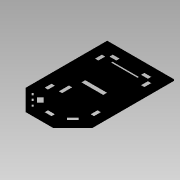
# Autodesk Inventor part: Base Kepala
Saved by Autodesk Inventor 2015 SP1 (Build 190203100, 203)
## iProperties
Created: 2015-02-13
Part Number: Base Kepala
Material: Generic
Document SubType Name: Modeling
Designer: Rafi Kurnia Putra
Density: 1 g/cm^3
Appearance: Default(1)
Author: Rafi Kurnia Putra
Autodesk Inventor part; units mm, degrees
ref_plane "YZ Plane" through (0, 0, 0) normal (1, 0, 0) x (0, 1, 0)
ref_plane "XZ Plane" through (0, 0, 0) normal (0, 1, 0) x (-1, 0, 0)
ref_plane "XY Plane" through (0, 0, 0) normal (0, 0, 1) x (1, 0, 0)
sketch "Sketch1" plane through (0, 0, 0) normal (0, 1, 0) x (-1, 0, 0)
  line L0 (31.6823, -78.8894) -> (44.0567, -66.5151)
  line L1 (24.6113, -71.8184) -> (31.6823, -78.8894)
  line L2 (36.9856, -59.444) -> (24.6113, -71.8184)
  line L3 (44.0567, -66.5151) -> (36.9856, -59.444)
  line L4 (8.75, -88.3884) -> (8.75, -78.3884)
  line L5 (-8.75, -88.3884) -> (8.75, -88.3884)
  line L6 (8.75, -78.3884) -> (-8.75, -78.3884)
  line L7 (-8.75, -78.3884) -> (-8.75, -88.3884)
  line L8 (-31.6827, -78.8894) -> (-24.6116, -71.8184)
  line L9 (-24.6116, -71.8184) -> (-36.986, -59.444)
  line L10 (-44.057, -66.5151) -> (-31.6827, -78.8894)
  line L11 (-36.986, -59.444) -> (-44.057, -66.5151)
  line L12 (-53.5557, -43.5826) -> (-43.5557, -43.5826)
  line L13 (-43.5557, -43.5826) -> (-43.5557, -26.0826)
  line L14 (-43.5557, -26.0826) -> (-53.5557, -26.0826)
  line L15 (-53.5557, -26.0826) -> (-53.5557, -43.5826)
  line L16 (-53.556, 80.1674) -> (-53.556, 62.6674)
  line L17 (-43.556, 80.1674) -> (-53.556, 80.1674)
  line L18 (-43.556, 62.6674) -> (-43.556, 80.1674)
  line L19 (-53.556, 62.6674) -> (-43.556, 62.6674)
  line L20 (-42.0848, 91.6386) -> (-42.0848, 81.6386)
  line L21 (-42.0848, 81.6386) -> (-24.5848, 81.6386)
  line L22 (-24.5848, 81.6386) -> (-24.5848, 91.6386)
  line L23 (-24.5848, 91.6386) -> (-42.0848, 91.6386)
  line L24 (42.0848, 91.6386) -> (24.5848, 91.6386)
  line L25 (42.0848, 81.6386) -> (42.0848, 91.6386)
  line L26 (24.5848, 81.6386) -> (42.0848, 81.6386)
  line L27 (24.5848, 91.6386) -> (24.5848, 81.6386)
  line L28 (43.556, 80.1674) -> (43.556, 62.6674)
  line L29 (53.556, 80.1674) -> (43.556, 80.1674)
  line L30 (53.556, 62.6674) -> (53.556, 80.1674)
  line L31 (43.556, 62.6674) -> (53.556, 62.6674)
  circle A0 centre (37.593, 75.6756) radius 1.75
  circle A1 centre (32.8575, 75.4371) radius 1.75
  circle A2 centre (50.5965, 88.6786) radius 1.75
  line L32 (29.3575, 78.4256) -> (-29.3575, 78.4256)
  line L33 (29.3575, 72.4486) -> (29.3575, 78.4256)
  line L34 (-29.3575, 72.4486) -> (29.3575, 72.4486)
  line L35 (-29.3575, 78.4256) -> (-29.3575, 72.4486)
  circle A3 centre (-32.8575, 75.4371) radius 1.75
  circle A4 centre (-37.593, 75.6756) radius 1.75
  circle A5 centre (-50.5965, 88.6786) radius 1.75
  line L36 (-24.5, 4.9331) -> (24.5, 4.9331)
  circle A6 centre (28, 4.9331) radius 1.75
  circle A7 centre (32.442, 26.7171) radius 1.5
  circle A8 centre (38, 31.4596) radius 1.75
  circle A9 centre (50.5965, 18.9376) radius 1.75
  circle A10 centre (32.4485, 53.6756) radius 1.75
  circle A11 centre (-32.4355, 53.6756) radius 1.75
  circle A12 centre (-50.5965, 18.9376) radius 1.75
  circle A13 centre (-32.442, 26.7171) radius 1.5
  circle A14 centre (-28, 4.9331) radius 1.75
  line L37 (-22.2, -10.9442) -> (-32, -10.9442)
  line L38 (-22.2, -35.1896) -> (-22.2, -10.9442)
  line L39 (-32, -35.1896) -> (-22.2, -35.1896)
  line L40 (-32, -10.9442) -> (-32, -35.1896)
  circle A15 centre (-49.906, -55.5042) radius 1.75
  circle A16 centre (-37.593, -48.9392) radius 1.75
  circle A17 centre (-20, -65.0669) radius 1.75
  circle A18 centre (13.2193, -19.3896) radius 1.75
  circle A19 centre (13.2193, -43.7996) radius 1.75
  circle A20 centre (20, -65.0669) radius 1.75
  circle A21 centre (37.593, -48.9392) radius 1.75
  circle A22 centre (39.7053, -43.7996) radius 1.75
  circle A23 centre (39.7053, -19.3896) radius 1.75
  circle A24 centre (49.9057, -55.5042) radius 1.75
  line L41 (43.5557, -43.5826) -> (53.5557, -43.5826)
  line L42 (43.5557, -26.0826) -> (43.5557, -43.5826)
  line L43 (53.5557, -26.0826) -> (43.5557, -26.0826)
  line L44 (53.5557, -43.5826) -> (53.5557, -26.0826)
  line L45 (24.5, 4.9331) -> (24.5, 15.9376)
  line L46 (24.5, 15.9376) -> (-24.5, 15.9376)
  line L47 (-24.5, 15.9376) -> (-24.5, 4.9331)
  circle A25 centre (14, 31.4596) radius 1.75
  circle A26 centre (-27.94, -53.8096) radius 1.75
  circle A27 centre (20.32, -47.4596) radius 1.75
  line L48 (70.4053, -63.9933) -> (29.1627, -105.2363)
  line L49 (29.1627, -105.2363) -> (-29.1634, -105.2362)
  line L50 (-29.1634, -105.2362) -> (-70.4063, -63.9936)
  line L51 (-70.4063, -63.9936) -> (-70.4063, 108.2408)
  line L52 (-70.4063, 108.2408) -> (70.4053, 108.2411)
  line L53 (70.4053, 108.2411) -> (70.4053, -63.9933)
  line L54 (37.7622, -79.6663) -> (44.8333, -72.5952)
  line L55 (44.8333, -72.5952) -> (46.9546, -74.7165)
  line L56 (46.9546, -74.7165) -> (39.8835, -81.7876)
  line L57 (39.8835, -81.7876) -> (37.7622, -79.6663)
  line L58 (37.7622, -79.6663) -> (46.9546, -74.7165) construction
  line L59 (44.8333, -72.5952) -> (39.8835, -81.7876) construction
  line L60 (34.2266, -83.2018) -> (27.1556, -90.2729)
  line L61 (27.1556, -90.2729) -> (29.2769, -92.3942)
  line L62 (29.2769, -92.3942) -> (36.348, -85.3231)
  line L63 (36.348, -85.3231) -> (34.2266, -83.2018)
  line L64 (34.2266, -83.2018) -> (29.2769, -92.3942) construction
  line L65 (27.1556, -90.2729) -> (36.348, -85.3231) construction
  line L66 (55.4401, -61.9888) -> (48.369, -69.0599)
  line L67 (48.369, -69.0599) -> (50.4903, -71.1812)
  line L68 (50.4903, -71.1812) -> (57.5614, -64.1101)
  line L69 (57.5614, -64.1101) -> (55.4401, -61.9888)
  line L70 (55.4401, -61.9888) -> (50.4903, -71.1812) construction
  line L71 (48.369, -69.0599) -> (57.5614, -64.1101) construction
  line L72 (5, -93.2363) -> (15, -93.2363) construction
  line L73 (-10, -93.2363) -> (-20, -93.2363)
  line L74 (-20, -93.2363) -> (-20, -96.2363)
  line L75 (-20, -96.2363) -> (-10, -96.2363)
  line L76 (-10, -96.2363) -> (-10, -93.2363)
  line L77 (-10, -93.2363) -> (-20, -96.2363) construction
  line L78 (-20, -93.2363) -> (-10, -96.2363) construction
  line L79 (-10, -93.2363) -> (0, -93.2363) construction
  line L80 (20, -96.237) -> (10, -96.237)
  line L81 (10, -96.237) -> (10, -93.237)
  line L82 (10, -93.237) -> (20, -93.237)
  line L83 (20, -93.237) -> (20, -96.237)
  line L84 (20, -96.237) -> (10, -93.237) construction
  line L85 (10, -96.237) -> (20, -93.237) construction
  line L86 (61.4053, 25.443) -> (61.4053, 10.443)
  line L87 (61.4053, 10.443) -> (58.4053, 10.443)
  line L88 (58.4053, 10.443) -> (58.4053, 25.443)
  line L89 (58.4053, 25.443) -> (61.4053, 25.443)
  line L90 (61.4053, 25.443) -> (58.4053, 10.443) construction
  line L91 (61.4053, 10.443) -> (58.4053, 25.443) construction
  line L92 (-37.8487, -79.5805) -> (-44.9198, -72.5095)
  line L93 (-44.9198, -72.5095) -> (-47.0411, -74.6308)
  line L94 (-47.0411, -74.6308) -> (-39.97, -81.7018)
  line L95 (-39.97, -81.7018) -> (-37.8487, -79.5805)
  line L96 (-37.8487, -79.5805) -> (-47.0411, -74.6308) construction
  line L97 (-34.3131, -83.116) -> (-27.242, -90.1871)
  line L98 (-27.242, -90.1871) -> (-29.3633, -92.3084)
  line L99 (-29.3633, -92.3084) -> (-36.4344, -85.2374)
  line L100 (-36.4344, -85.2374) -> (-34.3131, -83.116)
  line L101 (-34.3131, -83.116) -> (-29.3633, -92.3084) construction
  line L102 (-27.242, -90.1871) -> (-36.4344, -85.2374) construction
  line L103 (-55.5071, -61.8836) -> (-48.4359, -68.9546)
  line L104 (-48.4359, -68.9546) -> (-50.5766, -71.0953)
  line L105 (-50.5766, -71.0953) -> (-57.6477, -64.0243)
  line L106 (-57.6477, -64.0243) -> (-55.5071, -61.8836)
  line L107 (-55.5071, -61.8836) -> (-50.5766, -71.0953) construction
  line L108 (-48.4359, -68.9546) -> (-57.6477, -64.0243) construction
  line L109 (61.4053, -7.057) -> (61.4053, -22.057)
  line L110 (61.4053, -22.057) -> (58.4053, -22.057)
  line L111 (58.4053, -22.057) -> (58.4053, -7.057)
  line L112 (58.4053, -7.057) -> (61.4053, -7.057)
  line L113 (61.4053, -7.057) -> (58.4053, -22.057) construction
  line L114 (61.4053, -22.057) -> (58.4053, -7.057) construction
  line L115 (61.4053, -39.557) -> (61.4053, -54.557)
  line L116 (61.4053, -54.557) -> (58.4053, -54.557)
  line L117 (58.4053, -54.557) -> (58.4053, -39.557)
  line L118 (58.4053, -39.557) -> (61.4053, -39.557)
  line L119 (61.4053, -39.557) -> (58.4053, -54.557) construction
  line L120 (61.4053, -54.557) -> (58.4053, -39.557) construction
  line L121 (61.4053, 57.943) -> (61.4053, 42.943)
  line L122 (61.4053, 42.943) -> (58.4053, 42.943)
  line L123 (58.4053, 42.943) -> (58.4053, 57.943)
  line L124 (58.4053, 57.943) -> (61.4053, 57.943)
  line L125 (61.4053, 57.943) -> (58.4053, 42.943) construction
  line L126 (61.4053, 42.943) -> (58.4053, 57.943) construction
  line L127 (61.4053, 25.443) -> (61.4053, 10.443)
  line L128 (61.4053, 10.443) -> (58.4053, 10.443)
  line L129 (58.4053, 10.443) -> (58.4053, 25.443)
  line L130 (58.4053, 25.443) -> (61.4053, 25.443)
  line L131 (61.4053, 25.443) -> (58.4053, 10.443) construction
  line L132 (61.4053, 10.443) -> (58.4053, 25.443) construction
  line L133 (61.4053, -7.057) -> (61.4053, -22.057)
  line L134 (61.4053, -22.057) -> (58.4053, -22.057)
  line L135 (58.4053, -22.057) -> (58.4053, -7.057)
  line L136 (58.4053, -7.057) -> (61.4053, -7.057)
  line L137 (61.4053, -7.057) -> (58.4053, -22.057) construction
  line L138 (61.4053, -22.057) -> (58.4053, -7.057) construction
  line L139 (61.4053, 90.443) -> (61.4053, 75.443)
  line L140 (61.4053, 75.443) -> (58.4053, 75.443)
  line L141 (58.4053, 75.443) -> (58.4053, 90.443)
  line L142 (58.4053, 90.443) -> (61.4053, 90.443)
  line L143 (61.4053, 90.443) -> (58.4053, 75.443) construction
  line L144 (61.4053, 75.443) -> (58.4053, 90.443) construction
  line L145 (61.4053, 57.943) -> (61.4053, 42.943)
  line L146 (61.4053, 42.943) -> (58.4053, 42.943)
  line L147 (58.4053, 42.943) -> (58.4053, 57.943)
  line L148 (58.4053, 57.943) -> (61.4053, 57.943)
  line L149 (61.4053, 57.943) -> (58.4053, 42.943) construction
  line L150 (61.4053, 42.943) -> (58.4053, 57.943) construction
  line L151 (61.4053, 25.443) -> (61.4053, 10.443)
  line L152 (61.4053, 10.443) -> (58.4053, 10.443)
  line L153 (58.4053, 10.443) -> (58.4053, 25.443)
  line L154 (58.4053, 25.443) -> (61.4053, 25.443)
  line L155 (61.4053, 25.443) -> (58.4053, 10.443) construction
  line L156 (61.4053, 10.443) -> (58.4053, 25.443) construction
  line L157 (0, 0) -> (0, -22.057) construction
  line L158 (-61.4053, 25.443) -> (-61.4053, 10.443)
  line L159 (-61.4053, 10.443) -> (-58.4053, 10.443)
  line L160 (-58.4053, 10.443) -> (-58.4053, 25.443)
  line L161 (-58.4053, 25.443) -> (-61.4053, 25.443)
  line L162 (-61.4053, 25.443) -> (-58.4053, 10.443) construction
  line L163 (-61.4053, 10.443) -> (-58.4053, 25.443) construction
  line L164 (-58.4053, -7.057) -> (-61.4053, -7.057)
  line L165 (-58.4053, -22.057) -> (-58.4053, -7.057)
  line L166 (-61.4053, -22.057) -> (-58.4053, -22.057)
  line L167 (-61.4053, -7.057) -> (-61.4053, -22.057)
  line L168 (-61.4053, -7.057) -> (-58.4053, -22.057) construction
  line L169 (-61.4053, -22.057) -> (-58.4053, -7.057) construction
  line L170 (-58.4053, -39.557) -> (-61.4053, -39.557)
  line L171 (-58.4053, -54.557) -> (-58.4053, -39.557)
  line L172 (-61.4053, -54.557) -> (-58.4053, -54.557)
  line L173 (-61.4053, -39.557) -> (-61.4053, -54.557)
  line L174 (-61.4053, -39.557) -> (-58.4053, -54.557) construction
  line L175 (-61.4053, -54.557) -> (-58.4053, -39.557) construction
  line L176 (-58.4053, 57.943) -> (-61.4053, 57.943)
  line L177 (-58.4053, 42.943) -> (-58.4053, 57.943)
  line L178 (-61.4053, 42.943) -> (-58.4053, 42.943)
  line L179 (-61.4053, 57.943) -> (-61.4053, 42.943)
  line L180 (-61.4053, 57.943) -> (-58.4053, 42.943) construction
  line L181 (-61.4053, 42.943) -> (-58.4053, 57.943) construction
  line L182 (-58.4053, 25.443) -> (-61.4053, 25.443)
  line L183 (-58.4053, 10.443) -> (-58.4053, 25.443)
  line L184 (-61.4053, 10.443) -> (-58.4053, 10.443)
  line L185 (-61.4053, 25.443) -> (-61.4053, 10.443)
  line L186 (-61.4053, 25.443) -> (-58.4053, 10.443) construction
  line L187 (-61.4053, 10.443) -> (-58.4053, 25.443) construction
  line L188 (-58.4053, -7.057) -> (-61.4053, -7.057)
  line L189 (-58.4053, -22.057) -> (-58.4053, -7.057)
  line L190 (-61.4053, -22.057) -> (-58.4053, -22.057)
  line L191 (-61.4053, -7.057) -> (-61.4053, -22.057)
  line L192 (-61.4053, -7.057) -> (-58.4053, -22.057) construction
  line L193 (-61.4053, -22.057) -> (-58.4053, -7.057) construction
  line L194 (-58.4053, 90.443) -> (-61.4053, 90.443)
  line L195 (-58.4053, 75.443) -> (-58.4053, 90.443)
  line L196 (-61.4053, 75.443) -> (-58.4053, 75.443)
  line L197 (-61.4053, 90.443) -> (-61.4053, 75.443)
  line L198 (-61.4053, 90.443) -> (-58.4053, 75.443) construction
  line L199 (-61.4053, 75.443) -> (-58.4053, 90.443) construction
  line L200 (-58.4053, 57.943) -> (-61.4053, 57.943)
  line L201 (-58.4053, 42.943) -> (-58.4053, 57.943)
  line L202 (-61.4053, 42.943) -> (-58.4053, 42.943)
  line L203 (-61.4053, 57.943) -> (-61.4053, 42.943)
  line L204 (-61.4053, 57.943) -> (-58.4053, 42.943) construction
  line L205 (-61.4053, 42.943) -> (-58.4053, 57.943) construction
  line L206 (-58.4053, 25.443) -> (-61.4053, 25.443)
  line L207 (-58.4053, 10.443) -> (-58.4053, 25.443)
  line L208 (-61.4053, 10.443) -> (-58.4053, 10.443)
  line L209 (-61.4053, 25.443) -> (-61.4053, 10.443)
  line L210 (-61.4053, 25.443) -> (-58.4053, 10.443) construction
  line L211 (-61.4053, 10.443) -> (-58.4053, 25.443) construction
  line L212 (-7.5214, 96.2408) -> (7.4786, 96.2408)
  line L213 (7.4786, 96.2408) -> (7.4786, 99.2408)
  line L214 (7.4786, 99.2408) -> (-7.5214, 99.2408)
  line L215 (-7.5214, 99.2408) -> (-7.5214, 96.2408)
  line L216 (-7.5214, 96.2408) -> (7.4786, 99.2408) construction
  line L217 (7.4786, 96.2408) -> (-7.5214, 99.2408) construction
  line L218 (-30.5214, 96.2408) -> (-15.5214, 96.2408)
  line L219 (-15.5214, 96.2408) -> (-15.5214, 99.2408)
  line L220 (-15.5214, 99.2408) -> (-30.5214, 99.2408)
  line L221 (-30.5214, 99.2408) -> (-30.5214, 96.2408)
  line L222 (-30.5214, 96.2408) -> (-15.5214, 99.2408) construction
  line L223 (-15.5214, 96.2408) -> (-30.5214, 99.2408) construction
  line L224 (-53.5214, 96.2407) -> (-38.5214, 96.2407)
  line L225 (-38.5214, 96.2407) -> (-38.5214, 99.2407)
  line L226 (-38.5214, 99.2407) -> (-53.5214, 99.2407)
  line L227 (-53.5214, 99.2407) -> (-53.5214, 96.2407)
  line L228 (-53.5214, 96.2407) -> (-38.5214, 99.2407) construction
  line L229 (-38.5214, 96.2407) -> (-53.5214, 99.2407) construction
  line L230 (15.4786, 96.2409) -> (30.4786, 96.2409)
  line L231 (30.4786, 96.2409) -> (30.4786, 99.2409)
  line L232 (30.4786, 99.2409) -> (15.4786, 99.2409)
  line L233 (15.4786, 99.2409) -> (15.4786, 96.2409)
  line L234 (15.4786, 96.2409) -> (30.4786, 99.2409) construction
  line L235 (30.4786, 96.2409) -> (15.4786, 99.2409) construction
  line L236 (-7.5214, 96.2408) -> (7.4786, 96.2408)
  line L237 (7.4786, 96.2408) -> (7.4786, 99.2408)
  line L238 (7.4786, 99.2408) -> (-7.5214, 99.2408)
  line L239 (-7.5214, 99.2408) -> (-7.5214, 96.2408)
  line L240 (-7.5214, 96.2408) -> (7.4786, 99.2408) construction
  line L241 (7.4786, 96.2408) -> (-7.5214, 99.2408) construction
  line L242 (-30.5214, 96.2408) -> (-15.5214, 96.2408)
  line L243 (-15.5214, 96.2408) -> (-15.5214, 99.2408)
  line L244 (-15.5214, 99.2408) -> (-30.5214, 99.2408)
  line L245 (-30.5214, 99.2408) -> (-30.5214, 96.2408)
  line L246 (-30.5214, 96.2408) -> (-15.5214, 99.2408) construction
  line L247 (-15.5214, 96.2408) -> (-30.5214, 99.2408) construction
  line L248 (38.4786, 96.2409) -> (53.4786, 96.2409)
  line L249 (53.4786, 96.2409) -> (53.4786, 99.2409)
  line L250 (53.4786, 99.2409) -> (38.4786, 99.2409)
  line L251 (38.4786, 99.2409) -> (38.4786, 96.2409)
  line L252 (38.4786, 96.2409) -> (53.4786, 99.2409) construction
  line L253 (53.4786, 96.2409) -> (38.4786, 99.2409) construction
  line L254 (15.4786, 96.2409) -> (30.4786, 96.2409)
  line L255 (30.4786, 96.2409) -> (30.4786, 99.2409)
  line L256 (30.4786, 99.2409) -> (15.4786, 99.2409)
  line L257 (15.4786, 99.2409) -> (15.4786, 96.2409)
  line L258 (15.4786, 96.2409) -> (30.4786, 99.2409) construction
  line L259 (30.4786, 96.2409) -> (15.4786, 99.2409) construction
  line L260 (-7.5214, 96.2408) -> (7.4786, 96.2408)
  line L261 (7.4786, 96.2408) -> (7.4786, 99.2408)
  line L262 (7.4786, 99.2408) -> (-7.5214, 99.2408)
  line L263 (-7.5214, 99.2408) -> (-7.5214, 96.2408)
  line L264 (-7.5214, 96.2408) -> (7.4786, 99.2408) construction
  line L265 (7.4786, 96.2408) -> (-7.5214, 99.2408) construction
  point P0 (42.3584, -77.1914)
  point P1 (31.7518, -87.798)
  point P2 (52.9652, -66.585)
  point P3 (-15, -94.7363)
  point P4 (15, -94.737)
  point P5 (59.9053, 17.943)
  point P6 (-31.8382, -87.7122)
  point P7 (-53.0418, -66.4894)
  point P8 (-65.5064, -62.0457)
  point P9 (59.9053, -14.557)
  point P10 (59.9053, -47.057)
  point P11 (59.9053, 50.443)
  point P12 (59.9053, 17.943)
  point P13 (59.9053, -14.557)
  point P14 (59.9053, 82.943)
  point P15 (59.9053, 50.443)
  point P16 (59.9053, 17.943)
  point P17 (-0.0214, 97.7408)
  point P18 (-23.0214, 97.7408)
  point P19 (-46.0214, 97.7407)
  point P20 (22.9786, 97.7409)
  point P21 (-0.0214, 97.7408)
  point P22 (-23.0214, 97.7408)
  point P23 (45.9786, 97.7409)
  point P24 (22.9786, 97.7409)
  point P25 (-0.0214, 97.7408)
  dimension "d106" = 23
  dimension "d109" = 23
  dimension "d121" = 172.2345
  dimension "d122" = 140.8117
  dimension "d123" = 172.2345
  dimension "d124" = 58.3261
  dimension "d125" = 58.3261
  dimension "d126" = 58.3261
  dimension "d127" = 135
  dimension "d128" = 135
  dimension "d129" = 135
  dimension "d130" = 135
  dimension "d131" = 90
  dimension "d132" = 90
  dimension "d134" = 8.9994
  dimension "d135" = 8.9999
  dimension "d138" = 9
  dimension "d146" = 3
  dimension "d147" = 3
  dimension "d148" = 3
  dimension "d152" = 3
  dimension "d153" = 3
  dimension "d154" = 3
  dimension "d158" = 3
  dimension "d184" = 15
  dimension "d185" = 3
  dimension "d188" = 23
  dimension "d191" = 23
  constraints: 532 end point, 50 midpoint, 36 symmetric about line, 28 centre point, 17 parallel, 8 perpendicular, 7 horizontal, 3 collinear, 3 vertical, 2 coincident, 98 other
  measures "d121" distance of L52.end L48.start
  measures "d122" distance of L51.end L52.end
  measures "d123" distance of L50.end L51.end
  measures "d124" distance of L48.end L49.end
  measures "d125" distance of L48.start L48.end
  measures "d126" distance of L49.end L50.end
  measures "d127" angle of L48 L53
  measures "d128" angle of L49 L48
  measures "d129" angle of L49 L50
  measures "d130" angle of L50 L51
  measures "d131" angle of L52 L51
  measures "d132" angle of L53 L52
  measures "d134" distance from line of L48.end L80
  measures "d135" distance from line of L49.end L75
  measures "d138" distance from line of L49.end L94
  measures "d146" distance of L75.end L73.start
  measures "d147" distance of L80.end L81.end
  measures "d148" distance of L98.start L98.end
  measures "d152" distance of L60.end L61.end
  measures "d153" distance of L56.end L54.start
  measures "d154" distance of L66.end L67.end
  measures "d158" distance between parallel lines of L86 L88
  measures "d184" distance of L214.end L213.end
  measures "d185" distance of L213.end L212.end
  measures "d188" distance of L212.start L221.end
  measures "d191" distance of L212.start L233.end
extrude "Extrusion3" add sketch "Sketch1" along normal blind 3
body "Solid3"
